Autodesk Fusion 360 part; units mm, degrees
(part 2 of 2)
  spline S289 degree 3 poles (-117.5026, -9.5657) (-117.4851, -9.5569) (-117.4675, -9.5437) (-117.4499, -9.5261) knots 0 0 0 0 1 1 1 1
  spline S290 degree 3 poles (-119.0451, -14.0876) (-119.0187, -13.8591) (-118.9792, -13.6393) (-118.9265, -13.4284) knots 0 0 0 0 1 1 1 1
  line L134 (-80.6655, -26.5854) -> (-81.061, -26.9809)
  spline S291 degree 3 poles (-82.8276, -8.4187) (-82.8627, -8.4187) (-82.9375, -8.3967) (-83.0517, -8.3528) knots 0 0 0 0 1 1 1 1
  line L135 (-81.1665, -9.3679) -> (-82.8276, -8.4187)
  line L136 (-88.7601, -9.2361) -> (-87.9691, -8.7087)
  spline S292 degree 3 poles (-77.8706, -7.575) (-76.6402, -8.4539) (-75.5152, -9.5876) (-74.4957, -10.9763) knots 0 0 0 0 1 1 1 1
  spline S293 degree 3 poles (-118.3332, -11.1081) (-118.0783, -10.3874) (-117.819, -9.8865) (-117.5554, -9.6052) knots 0 0 0 0 1 1 1 1
  line L137 (-77.2115, -23.2368) -> (-80.6655, -26.5854)
  line L138 (-81.7466, -5.9666) -> (-81.6806, -5.9666)
  spline S294 degree 3 poles (-79.9141, -6.4017) (-79.2549, -6.6917) (-78.5738, -7.0828) (-77.8706, -7.575) knots 0 0 0 0 1 1 1 1
  spline S295 degree 3 poles (-81.6147, -5.9666) (-81.1401, -5.9666) (-80.5732, -6.1116) (-79.9141, -6.4017) knots 0 0 0 0 1 1 1 1
  spline S296 degree 3 poles (-72.9664, -15.3795) (-72.9664, -16.4166) (-73.2037, -17.423) (-73.6783, -18.3985) knots 0 0 0 0 1 1 1 1
  line L139 (-92.4251, -25.9262) -> (-92.4251, -21.8921)
  line L140 (-92.4251, -21.8921) -> (-92.4251, -8.3923)
  line L141 (-81.6806, -5.9666) -> (-81.6147, -5.9666)
  spline S297 degree 3 poles (-86.4135, -7.8123) (-85.5522, -7.3377) (-84.7216, -6.9378) (-83.9218, -6.6126) knots 0 0 0 0 1 1 1 1
  spline S298 degree 3 poles (-98.9405, -9.4998) (-99.0108, -9.6052) (-99.0987, -9.7107) (-99.2041, -9.8162) knots 0 0 0 0 1 1 1 1
  spline S299 degree 3 poles (-98.69, -9.1306) (-98.7515, -9.2537) (-98.835, -9.3767) (-98.9405, -9.4998) knots 0 0 0 0 1 1 1 1
  spline S300 degree 3 poles (-76.7896, -16.3024) (-76.7896, -15.1422) (-77.0884, -14.0568) (-77.6861, -13.0461) knots 0 0 0 0 1 1 1 1
  line L142 (-98.5977, -8.7351) -> (-98.5977, -8.7615)
  arc A32 (-108.5643, -6.5335) -> (-108.3534, -6.5467) centre (-108.3531, -4.8477) ccw
  spline S301 degree 3 poles (-112.0711, -8.4714) (-112.4051, -8.4714) (-112.7215, -8.4934) (-113.0203, -8.5374) knots 0 0 0 0 1 1 1 1
  spline S302 degree 3 poles (-104.2665, -9.2625) (-104.3544, -9.2449) (-104.4423, -9.2361) (-104.5302, -9.2361) knots 0 0 0 0 1 1 1 1
  spline S303 degree 3 poles (-101.4321, -11.0422) (-101.4936, -10.8225) (-101.5947, -10.5984) (-101.7353, -10.3699) knots 0 0 0 0 1 1 1 1
  spline S304 degree 3 poles (-110.2518, -8.5769) (-110.5682, -8.5593) (-110.8758, -8.5374) (-111.1746, -8.511) knots 0 0 0 0 1 1 1 1
  line L143 (-76.7896, -16.3683) -> (-76.7896, -16.3024)
  line L144 (-88.7601, -6.573) -> (-88.7601, -9.2361)
  spline S305 degree 3 poles (-119.111, -14.7467) (-119.0934, -14.5358) (-119.0715, -14.3161) (-119.0451, -14.0876) knots 0 0 0 0 1 1 1 1
  spline S306 degree 3 poles (-73.6783, -18.3985) (-74.1529, -19.3741) (-74.6803, -20.2486) (-75.2603, -21.022) knots 0 0 0 0 1 1 1 1
  line L145 (-108.3534, -6.5467) -> (-102.3418, -7.1531)
  spline S307 degree 3 poles (-101.3926, -12.1892) (-101.3574, -12.031) (-101.3398, -11.8728) (-101.3398, -11.7146) knots 0 0 0 0 1 1 1 1
  line L146 (-92.4251, -8.3923) -> (-97.092, -8.3132)
  line L147 (-99.2041, -9.8162) -> (-99.5205, -10.1326)
  spline S308 degree 3 poles (-83.0517, -8.3528) (-83.166, -8.3089) (-83.311, -8.2605) (-83.4868, -8.2078) knots 0 0 0 0 1 1 1 1
  spline S309 degree 3 poles (-104.5302, -9.2361) (-104.6181, -9.2361) (-104.706, -9.2273) (-104.7939, -9.2097) knots 0 0 0 0 1 1 1 1
  line L148 (-100.7598, -11.6882) -> (-100.7861, -11.7146)
  line L149 (-125.9672, -11.385) -> (-125.9672, -11.3191)
  spline S310 degree 3 poles (-101.5508, -12.6901) (-101.4804, -12.5144) (-101.4277, -12.3474) (-101.3926, -12.1892) knots 0 0 0 0 1 1 1 1
  spline S311 degree 3 poles (-101.1553, -12.1892) (-101.2783, -12.3474) (-101.4101, -12.5144) (-101.5508, -12.6901) knots 0 0 0 0 1 1 1 1
  line L150 (-100.7861, -11.7146) -> (-101.1553, -12.1892)
  arc A33 (-166.7633, -25.979) -> (-166.961, -26.0317) centre (-165.2752, -31.9564) ccw
  spline S312 degree 3 poles (-99.9951, -10.6599) (-100.1357, -10.8532) (-100.2632, -11.0246) (-100.3774, -11.174) knots 0 0 0 0 1 1 1 1
  line L151 (-185.9055, -15.2345) -> (-185.9055, -15.2477)
  spline S313 degree 3 poles (-179.9203, -26.4272) (-180.0433, -26.4272) (-180.1708, -26.4228) (-180.3026, -26.414) knots 0 0 0 0 1 1 1 1
  spline S314 degree 3 poles (-187.7644, -20.9693) (-188.6872, -19.7564) (-189.2277, -18.5172) (-189.3859, -17.2516) knots 0 0 0 0 1 1 1 1
  spline S315 degree 3 poles (-175.2534, -7.3377) (-175.2006, -7.3201) (-175.1523, -7.2937) (-175.1084, -7.2586) knots 0 0 0 0 1 1 1 1
  spline S316 degree 3 poles (-189.3859, -17.2516) (-189.4035, -17.1637) (-189.4167, -17.0802) (-189.4255, -17.0011) knots 0 0 0 0 1 1 1 1
  line L152 (-172.3003, -8.7087) -> (-177.0463, -8.656)
  spline S317 degree 3 poles (-166.2623, -25.7417) (-166.3326, -25.7944) (-166.4073, -25.8383) (-166.4864, -25.8735) knots 0 0 0 0 1 1 1 1
  spline S318 degree 3 poles (-99.5205, -10.1326) (-99.6084, -10.2204) (-99.6919, -10.3083) (-99.771, -10.3962) knots 0 0 0 0 1 1 1 1
  line L153 (-186.5911, -10.1853) -> (-185.721, -8.6824)
  spline S319 degree 3 poles (-166.4864, -25.8735) (-166.5655, -25.9087) (-166.6578, -25.9438) (-166.7633, -25.979) knots 0 0 0 0 1 1 1 1
  spline S320 degree 3 poles (-99.7578, -15.3268) (-99.8809, -15.3971) (-100.0479, -15.4894) (-100.2588, -15.6037) knots 0 0 0 0 1 1 1 1
  line L154 (-99.8106, -15.1159) -> (-99.7578, -15.3268)
  spline S321 degree 3 poles (-100.2588, -15.6037) (-100.4697, -15.7179) (-100.707, -15.8278) (-100.9707, -15.9332) knots 0 0 0 0 1 1 1 1
  line L155 (-167.6597, -26.0581) -> (-172.2212, -25.979)
  spline S322 degree 3 poles (-186.7493, -10.4226) (-186.7141, -10.3874) (-186.6834, -10.3479) (-186.657, -10.3039) knots 0 0 0 0 1 1 1 1
  spline S323 degree 3 poles (-188.1994, -7.074) (-187.8127, -6.8982) (-187.593, -6.8016) (-187.5403, -6.784) knots 0 0 0 0 1 1 1 1
  line L156 (-185.721, -8.6824) -> (-190.757, -8.6033)
  spline S324 degree 3 poles (-99.771, -10.3962) (-99.8501, -10.4841) (-99.9248, -10.572) (-99.9951, -10.6599) knots 0 0 0 0 1 1 1 1
  line L157 (-177.0463, -8.656) -> (-175.2534, -7.3377)
  spline S325 degree 3 poles (-175.9916, -25.4253) (-176.6596, -25.7592) (-177.3276, -26.0097) (-177.9955, -26.1767) knots 0 0 0 0 1 1 1 1
  line L158 (-172.3003, -22.1294) -> (-172.3003, -8.7087)
  line L159 (-172.2212, -23.2896) -> (-174.9633, -24.8716)
  line L160 (-172.4321, -22.4195) -> (-172.3003, -22.1294)
  spline S326 degree 3 poles (-179.683, -22.8677) (-179.0326, -23.2193) (-178.3822, -23.4961) (-177.7318, -23.6982) knots 0 0 0 0 1 1 1 1
  spline S327 degree 3 poles (-177.7318, -23.6982) (-177.0815, -23.9004) (-176.4838, -24.0015) (-175.9389, -24.0015) knots 0 0 0 0 1 1 1 1
  spline S328 degree 3 poles (-166.961, -26.0317) (-167.0225, -26.0493) (-167.0797, -26.0581) (-167.1324, -26.0581) knots 0 0 0 0 1 1 1 1
  spline S329 degree 3 poles (-189.465, -7.7332) (-189.008, -7.4695) (-188.5862, -7.2498) (-188.1994, -7.074) knots 0 0 0 0 1 1 1 1
  spline S330 degree 3 poles (-190.1506, -8.155) (-189.9221, -7.9968) (-189.6936, -7.8562) (-189.465, -7.7332) knots 0 0 0 0 1 1 1 1
  line L161 (-189.4387, -16.6979) -> (-189.4387, -16.6451)
  line L162 (-189.4387, -16.777) -> (-189.4387, -16.6979)
  spline S331 degree 3 poles (-100.7334, -11.6355) (-100.7334, -11.653) (-100.7422, -11.6706) (-100.7598, -11.6882) knots 0 0 0 0 1 1 1 1
  spline S332 degree 3 poles (-180.7113, -26.3745) (-181.1332, -26.3217) (-181.7132, -26.0932) (-182.4515, -25.6889) knots 0 0 0 0 1 1 1 1
  spline S333 degree 3 poles (-189.4387, -16.6451) (-189.4387, -15.6608) (-189.1574, -14.6588) (-188.5949, -13.6393) knots 0 0 0 0 1 1 1 1
  spline S334 degree 3 poles (-184.7454, -24.1069) (-185.8352, -23.228) (-186.8416, -22.1822) (-187.7644, -20.9693) knots 0 0 0 0 1 1 1 1
  arc A34 (-100.7334, -11.6355) -> (-100.3774, -11.174) centre (-156.8917, 32.0547) ccw
  spline S335 degree 3 poles (-177.9955, -26.1767) (-178.6635, -26.3437) (-179.3051, -26.4272) (-179.9203, -26.4272) knots 0 0 0 0 1 1 1 1
  line L163 (-185.9055, -15.195) -> (-185.9055, -15.2345)
  spline S336 degree 3 poles (-174.9633, -24.8716) (-175.1391, -24.9946) (-175.3105, -25.1001) (-175.4775, -25.188) knots 0 0 0 0 1 1 1 1
  line L164 (-167.5015, -26.0581) -> (-167.5675, -26.0581)
  spline S337 degree 3 poles (-186.657, -10.3039) (-186.6306, -10.26) (-186.6086, -10.2204) (-186.5911, -10.1853) knots 0 0 0 0 1 1 1 1
  line L165 (-185.9055, -15.2477) -> (-185.9055, -15.2213)
  spline S338 degree 3 poles (-100.9707, -15.9332) (-101.1816, -16.0387) (-101.4057, -16.1354) (-101.643, -16.2233) knots 0 0 0 0 1 1 1 1
  spline S339 degree 3 poles (-180.3026, -26.414) (-180.4344, -26.4052) (-180.5707, -26.3921) (-180.7113, -26.3745) knots 0 0 0 0 1 1 1 1
  line L166 (-167.5675, -26.0581) -> (-167.6597, -26.0581)
  spline S340 degree 3 poles (-188.5949, -13.6393) (-188.0325, -12.6198) (-187.4172, -11.5476) (-186.7493, -10.4226) knots 0 0 0 0 1 1 1 1
  spline S341 degree 3 poles (-189.4255, -17.0011) (-189.4343, -16.922) (-189.4387, -16.8473) (-189.4387, -16.777) knots 0 0 0 0 1 1 1 1
  line L167 (-172.2212, -25.979) -> (-172.2212, -23.2896)
  line L168 (-167.317, -26.0581) -> (-167.5015, -26.0581)
  arc A35 (-175.9916, -25.4253) -> (-175.4775, -25.188) centre (-178.0133, -20.3693) ccw
  arc A36 (-102.3681, -16.4606) -> (-101.643, -16.2233) centre (-105.1088, -6.8599) ccw
  spline S342 degree 3 poles (-175.1084, -7.2586) (-175.0644, -7.2234) (-175.0161, -7.1883) (-174.9633, -7.1531) knots 0 0 0 0 1 1 1 1
  spline S343 degree 3 poles (-172.9858, -23.0786) (-172.7046, -22.8325) (-172.52, -22.6128) (-172.4321, -22.4195) knots 0 0 0 0 1 1 1 1
  spline S344 degree 3 poles (-182.4515, -25.6889) (-183.1898, -25.2846) (-183.9544, -24.7573) (-184.7454, -24.1069) knots 0 0 0 0 1 1 1 1
  spline S345 degree 3 poles (-190.757, -8.6033) (-190.5812, -8.4627) (-190.3791, -8.3132) (-190.1506, -8.155) knots 0 0 0 0 1 1 1 1
  line L169 (-167.1324, -26.0581) -> (-167.317, -26.0581)
  line L170 (-175.9389, -24.0015) -> (-175.8862, -24.0015)
  spline S346 degree 3 poles (-174.0141, -23.6719) (-173.5747, -23.4873) (-173.2319, -23.2896) (-172.9858, -23.0786) knots 0 0 0 0 1 1 1 1
  line L171 (-175.7807, -24.0015) -> (-175.728, -24.0015)
  line L172 (-175.8862, -24.0015) -> (-175.8334, -24.0015)
  spline S347 degree 3 poles (-175.728, -24.0015) (-175.0249, -23.9663) (-174.4536, -23.8564) (-174.0141, -23.6719) knots 0 0 0 0 1 1 1 1
  line L173 (-175.8334, -24.0015) -> (-175.7807, -24.0015)
  spline S348 degree 3 poles (-183.4007, -20.1124) (-182.2406, -21.2637) (-181.0013, -22.1822) (-179.683, -22.8677) knots 0 0 0 0 1 1 1 1
  spline S349 degree 3 poles (-174.9633, -7.1531) (-174.8754, -7.1004) (-174.7832, -7.0476) (-174.6865, -6.9949) knots 0 0 0 0 1 1 1 1
  line L174 (-173.4341, -6.7049) -> (-168.6353, -6.6785)
  arc A37 (-174.3833, -6.8631) -> (-174.6865, -6.9949) centre (-173.796, -8.6285) ccw
  line L175 (-200.4961, -12.2155) -> (-200.4961, -12.0573)
  spline S350 degree 3 poles (-173.9614, -6.7576) (-173.8911, -6.74) (-173.812, -6.7268) (-173.7241, -6.7181) knots 0 0 0 0 1 1 1 1
  spline S351 degree 3 poles (-206.6263, -17.067) (-206.5824, -17.0494) (-206.5428, -17.0319) (-206.5077, -17.0143) knots 0 0 0 0 1 1 1 1
  spline S352 degree 3 poles (-207.5887, -8.1814) (-207.7469, -8.199) (-207.9095, -8.2254) (-208.0765, -8.2605) knots 0 0 0 0 1 1 1 1
  spline S353 degree 3 poles (-166.17, -25.6889) (-166.1964, -25.7065) (-166.2271, -25.7241) (-166.2623, -25.7417) knots 0 0 0 0 1 1 1 1
  spline S354 degree 3 poles (-205.1762, -16.5265) (-205.0619, -16.4825) (-204.952, -16.4342) (-204.8466, -16.3815) knots 0 0 0 0 1 1 1 1
  spline S355 degree 3 poles (-206.6, -8.1814) (-206.6439, -8.1814) (-206.6835, -8.1726) (-206.7186, -8.155) knots 0 0 0 0 1 1 1 1
  spline S356 degree 3 poles (-200.4961, -12.0573) (-200.4961, -12.0046) (-200.5049, -11.9606) (-200.5224, -11.9255) knots 0 0 0 0 1 1 1 1
  spline S357 degree 3 poles (-195.2623, -25.1616) (-195.4293, -25.2671) (-195.5918, -25.3637) (-195.75, -25.4516) knots 0 0 0 0 1 1 1 1
  spline S358 degree 3 poles (-166.1041, -25.6098) (-166.1217, -25.645) (-166.1437, -25.6714) (-166.17, -25.6889) knots 0 0 0 0 1 1 1 1
  spline S359 degree 3 poles (-202.8954, -15.2609) (-202.2626, -14.8127) (-201.7441, -14.3512) (-201.3398, -13.8766) knots 0 0 0 0 1 1 1 1
  spline S360 degree 3 poles (-206.745, -17.1197) (-206.7098, -17.1022) (-206.6703, -17.0846) (-206.6263, -17.067) knots 0 0 0 0 1 1 1 1
  spline S361 degree 3 poles (-207.2855, -8.1682) (-207.3822, -8.177) (-207.4833, -8.1814) (-207.5887, -8.1814) knots 0 0 0 0 1 1 1 1
  spline S362 degree 3 poles (-208.0765, -8.2605) (-208.2435, -8.2957) (-208.4237, -8.3308) (-208.617, -8.366) knots 0 0 0 0 1 1 1 1
  spline S363 degree 3 poles (-195.75, -25.4516) (-196.0664, -25.6098) (-196.3916, -25.7417) (-196.7256, -25.8471) knots 0 0 0 0 1 1 1 1
  spline S364 degree 3 poles (-193.878, -24.397) (-194.0362, -24.4849) (-194.1856, -24.564) (-194.3262, -24.6343) knots 0 0 0 0 1 1 1 1
  line L176 (-164.2321, -24.186) -> (-166.1041, -25.6098)
  arc A38 (-194.7481, -24.8716) -> (-195.2623, -25.1616) centre (-192.0994, -30.1677) ccw
  spline S365 degree 3 poles (-205.5057, -16.6188) (-205.4003, -16.6012) (-205.2904, -16.5704) (-205.1762, -16.5265) knots 0 0 0 0 1 1 1 1
  spline S366 degree 3 poles (-205.5848, -19.3082) (-205.954, -18.8687) (-206.2836, -18.4601) (-206.5736, -18.0821) knots 0 0 0 0 1 1 1 1
  spline S367 degree 3 poles (-207.035, -17.3307) (-207.0174, -17.2779) (-206.9823, -17.234) (-206.9296, -17.1988) knots 0 0 0 0 1 1 1 1
  line L177 (-206.5077, -17.0143) -> (-205.5057, -16.6188)
  spline S368 degree 3 poles (-192.5333, -23.3555) (-192.3927, -23.2764) (-192.3136, -23.2368) (-192.296, -23.2368) knots 0 0 0 0 1 1 1 1
  spline S369 degree 3 poles (-204.8466, -16.3815) (-204.1786, -16.0827) (-203.5282, -15.7091) (-202.8954, -15.2609) knots 0 0 0 0 1 1 1 1
  spline S370 degree 3 poles (-194.3262, -24.6343) (-194.4669, -24.7046) (-194.6075, -24.7837) (-194.7481, -24.8716) knots 0 0 0 0 1 1 1 1
  spline S371 degree 3 poles (-185.8528, -15.9332) (-185.8176, -16.1442) (-185.7737, -16.3463) (-185.721, -16.5397) knots 0 0 0 0 1 1 1 1
  line L178 (-185.9055, -15.2213) -> (-185.9319, -15.3004)
  line L179 (-168.5035, -24.0278) -> (-164.2321, -24.186)
  spline S372 degree 3 poles (-205.5189, -19.3873) (-205.5453, -19.3521) (-205.5673, -19.3258) (-205.5848, -19.3082) knots 0 0 0 0 1 1 1 1
  spline S373 degree 3 poles (-206.5736, -18.0821) (-206.8636, -17.7042) (-207.0174, -17.4625) (-207.035, -17.357) knots 0 0 0 0 1 1 1 1
  line L180 (-206.8636, -8.155) -> (-206.9823, -8.155)
  spline S374 degree 3 poles (-202.7109, -9.1438) (-203.8534, -8.5725) (-205.1015, -8.2517) (-206.4549, -8.1814) knots 0 0 0 0 1 1 1 1
  line L181 (-192.296, -23.2368) -> (-192.1114, -23.5532)
  line L182 (-206.4549, -8.1814) -> (-206.6, -8.1814)
  line L183 (-174.3833, -6.8631) -> (-174.1723, -6.8103)
  spline S375 degree 3 poles (-200.5224, -11.9255) (-200.8388, -10.6423) (-201.5683, -9.7151) (-202.7109, -9.1438) knots 0 0 0 0 1 1 1 1
  spline S376 degree 3 poles (-196.7256, -25.8471) (-197.0596, -25.9526) (-197.4287, -26.0053) (-197.833, -26.0053) knots 0 0 0 0 1 1 1 1
  line L184 (-192.1114, -23.5532) -> (-193.878, -24.397)
  line L185 (-168.6353, -6.6785) -> (-168.5826, -10.5281)
  line L186 (-168.5826, -10.5281) -> (-168.5035, -24.0278)
  spline S377 degree 3 poles (-206.9823, -8.155) (-207.0878, -8.155) (-207.1888, -8.1594) (-207.2855, -8.1682) knots 0 0 0 0 1 1 1 1
  spline S378 degree 3 poles (-193.0606, -23.606) (-192.8497, -23.5181) (-192.6739, -23.4346) (-192.5333, -23.3555) knots 0 0 0 0 1 1 1 1
  spline S379 degree 3 poles (-173.7241, -6.7181) (-173.6362, -6.7093) (-173.5395, -6.7049) (-173.4341, -6.7049) knots 0 0 0 0 1 1 1 1
  spline S380 degree 3 poles (-206.9296, -17.1988) (-206.8768, -17.1637) (-206.8153, -17.1373) (-206.745, -17.1197) knots 0 0 0 0 1 1 1 1
  spline S381 degree 3 poles (-186.2483, -6.6785) (-186.0549, -6.6785) (-185.8484, -6.6829) (-185.6287, -6.6917) knots 0 0 0 0 1 1 1 1
  spline S382 degree 3 poles (-185.6287, -6.6917) (-185.409, -6.7005) (-185.1848, -6.7049) (-184.9563, -6.7049) knots 0 0 0 0 1 1 1 1
  spline S383 degree 3 poles (-187.0129, -6.7049) (-186.7844, -6.6873) (-186.5295, -6.6785) (-186.2483, -6.6785) knots 0 0 0 0 1 1 1 1
  spline S384 degree 3 poles (-153.2463, -6.4148) (-152.9739, -6.4324) (-152.6883, -6.4588) (-152.3894, -6.4939) knots 0 0 0 0 1 1 1 1
  spline S385 degree 3 poles (-187.5403, -6.784) (-187.4172, -6.7488) (-187.2415, -6.7225) (-187.0129, -6.7049) knots 0 0 0 0 1 1 1 1
  spline S386 degree 3 poles (-200.7202, -13.0197) (-200.5708, -12.7297) (-200.4961, -12.4616) (-200.4961, -12.2155) knots 0 0 0 0 1 1 1 1
  spline S387 degree 3 poles (-185.721, -16.5397) (-185.3343, -17.7701) (-184.5608, -18.961) (-183.4007, -20.1124) knots 0 0 0 0 1 1 1 1
  line L187 (-206.7186, -8.155) -> (-206.8636, -8.155)
  line L188 (-154.2483, -6.3885) -> (-153.9978, -6.3885)
  spline S388 degree 3 poles (-153.9978, -6.3885) (-153.7693, -6.3885) (-153.5188, -6.3973) (-153.2463, -6.4148) knots 0 0 0 0 1 1 1 1
  spline S389 degree 3 poles (-154.4724, -6.4148) (-154.4021, -6.3973) (-154.3274, -6.3885) (-154.2483, -6.3885) knots 0 0 0 0 1 1 1 1
  line L189 (-174.1723, -6.8103) -> (-173.9614, -6.7576)
  line L190 (-207.035, -17.357) -> (-207.035, -17.3307)
  line L191 (-197.833, -26.0053) -> (-197.8989, -26.0053)
  spline S390 degree 3 poles (-201.3398, -13.8766) (-201.0761, -13.5954) (-200.8696, -13.3097) (-200.7202, -13.0197) knots 0 0 0 0 1 1 1 1
  arc A39 (-185.9319, -15.3004) -> (-185.8528, -15.9332) centre (-178.1834, -14.6532) ccw
  line L192 (-208.617, -8.366) -> (-208.617, -8.3396)
  spline S391 degree 3 poles (-146.2196, -16.5133) (-147.1688, -16.7242) (-148.1664, -16.8649) (-149.2122, -16.9352) knots 0 0 0 0 1 1 1 1
  spline S392 degree 3 poles (-143.873, -15.6037) (-144.0839, -15.7179) (-144.3212, -15.8278) (-144.5849, -15.9332) knots 0 0 0 0 1 1 1 1
  line L193 (-143.4247, -15.1159) -> (-143.372, -15.3268)
  arc A40 (-144.3476, -11.6355) -> (-143.9916, -11.174) centre (-200.5059, 32.0547) ccw
  line L194 (-142.8183, -9.8162) -> (-143.1347, -10.1326)
  spline S393 degree 3 poles (-145.3495, -10.3699) (-145.6132, -9.9128) (-145.9735, -9.6228) (-146.4305, -9.4998) knots 0 0 0 0 1 1 1 1
  line L195 (-144.3739, -11.6882) -> (-144.4003, -11.7146)
  spline S394 degree 3 poles (-145.2968, -7.2586) (-144.9276, -7.3113) (-144.5233, -7.3992) (-144.0839, -7.5222) knots 0 0 0 0 1 1 1 1
  arc A41 (-184.7981, -11.5564) -> (-184.429, -10.8049) centre (-238.7282, 15.402) ccw
  line L196 (-144.4003, -11.7146) -> (-144.7694, -12.1892)
  spline S395 degree 3 poles (-158.6647, -8.6824) (-158.4538, -8.6121) (-158.2428, -8.533) (-158.0319, -8.4451) knots 0 0 0 0 1 1 1 1
  line L197 (-185.9055, -15.1422) -> (-185.9055, -15.1554)
  spline S396 degree 3 poles (-185.576, -13.5207) (-185.7957, -14.1623) (-185.9055, -14.7028) (-185.9055, -15.1422) knots 0 0 0 0 1 1 1 1
  spline S397 degree 3 poles (-147.8807, -9.2625) (-147.9686, -9.2449) (-148.0565, -9.2361) (-148.1444, -9.2361) knots 0 0 0 0 1 1 1 1
  spline S398 degree 3 poles (-155.6853, -8.4714) (-156.0193, -8.4714) (-156.3357, -8.4934) (-156.6345, -8.5374) knots 0 0 0 0 1 1 1 1
  spline S399 degree 3 poles (-145.9823, -16.4606) (-146.0175, -16.4606) (-146.057, -16.465) (-146.101, -16.4738) knots 0 0 0 0 1 1 1 1
  spline S400 degree 3 poles (-144.0839, -7.5222) (-143.6269, -7.6453) (-143.205, -7.8035) (-142.8183, -7.9968) knots 0 0 0 0 1 1 1 1
  spline S401 degree 3 poles (-156.2917, -7.4695) (-155.9402, -7.2234) (-155.6106, -6.9905) (-155.303, -6.7708) knots 0 0 0 0 1 1 1 1
  spline S402 degree 3 poles (-144.3476, -11.6355) (-144.3476, -11.653) (-144.3564, -11.6706) (-144.3739, -11.6882) knots 0 0 0 0 1 1 1 1
  spline S403 degree 3 poles (-158.5065, -17.1197) (-158.3132, -17.4361) (-158.0363, -17.8053) (-157.676, -18.2271) knots 0 0 0 0 1 1 1 1
  spline S404 degree 3 poles (-146.4305, -9.4998) (-146.8876, -9.3767) (-147.371, -9.2976) (-147.8807, -9.2625) knots 0 0 0 0 1 1 1 1
  spline S405 degree 3 poles (-184.7981, -11.5564) (-185.097, -12.2243) (-185.3562, -12.8791) (-185.576, -13.5207) knots 0 0 0 0 1 1 1 1
  spline S406 degree 3 poles (-144.5849, -15.9332) (-144.7958, -16.0387) (-145.0199, -16.1354) (-145.2572, -16.2233) knots 0 0 0 0 1 1 1 1
  spline S407 degree 3 poles (-158.0319, -8.4451) (-157.821, -8.3572) (-157.6188, -8.2693) (-157.4255, -8.1814) knots 0 0 0 0 1 1 1 1
  spline S408 degree 3 poles (-144.954, -11.7146) (-144.954, -11.486) (-144.9848, -11.2619) (-145.0463, -11.0422) knots 0 0 0 0 1 1 1 1
  spline S409 degree 3 poles (-182.1878, -6.9422) (-182.223, -6.9598) (-182.4295, -7.2762) (-182.8074, -7.8914) knots 0 0 0 0 1 1 1 1
  line L198 (-151.9676, -6.5467) -> (-145.9559, -7.1531)
  spline S410 degree 3 poles (-145.1649, -12.6901) (-145.0946, -12.5144) (-145.0419, -12.3474) (-145.0067, -12.1892) knots 0 0 0 0 1 1 1 1
  spline S411 degree 3 poles (-145.0463, -11.0422) (-145.1078, -10.8225) (-145.2089, -10.5984) (-145.3495, -10.3699) knots 0 0 0 0 1 1 1 1
  spline S412 degree 3 poles (-182.8074, -7.8914) (-183.1854, -8.5066) (-183.5941, -9.2361) (-184.0335, -10.0798) knots 0 0 0 0 1 1 1 1
  spline S413 degree 3 poles (-184.0335, -10.0798) (-184.1741, -10.3083) (-184.306, -10.55) (-184.429, -10.8049) knots 0 0 0 0 1 1 1 1
  arc A42 (-183.5062, -6.8103) -> (-184.2181, -6.7576) centre (-193.5222, -137.1956) ccw
  line L199 (-184.9563, -6.7049) -> (-184.2181, -6.7576)
  spline S414 degree 3 poles (-182.5965, -6.9026) (-182.3416, -6.929) (-182.2054, -6.9422) (-182.1878, -6.9422) knots 0 0 0 0 1 1 1 1
  spline S415 degree 3 poles (-142.8183, -7.9968) (-142.4316, -8.1902) (-142.2294, -8.4363) (-142.2119, -8.7351) knots 0 0 0 0 1 1 1 1
  arc A43 (-145.9823, -16.4606) -> (-145.2572, -16.2233) centre (-148.723, -6.8599) ccw
  spline S416 degree 3 poles (-142.5546, -9.4998) (-142.6249, -9.6052) (-142.7128, -9.7107) (-142.8183, -9.8162) knots 0 0 0 0 1 1 1 1
  line L200 (-161.0641, -9.4998) -> (-161.1168, -9.5261)
  spline S417 degree 3 poles (-143.372, -15.3268) (-143.495, -15.3971) (-143.662, -15.4894) (-143.873, -15.6037) knots 0 0 0 0 1 1 1 1
  spline S418 degree 3 poles (-142.2119, -8.7615) (-142.2119, -8.8845) (-142.2426, -9.0076) (-142.3041, -9.1306) knots 0 0 0 0 1 1 1 1
  spline S419 degree 3 poles (-148.1444, -9.2361) (-148.2323, -9.2361) (-148.3202, -9.2273) (-148.408, -9.2097) knots 0 0 0 0 1 1 1 1
  line L201 (-185.9055, -15.1554) -> (-185.9055, -15.195)
  spline S420 degree 3 poles (-143.8598, -15.2477) (-143.7279, -15.2125) (-143.5829, -15.1686) (-143.4247, -15.1159) knots 0 0 0 0 1 1 1 1
  spline S421 degree 3 poles (-143.3852, -10.3962) (-143.4643, -10.4841) (-143.539, -10.572) (-143.6093, -10.6599) knots 0 0 0 0 1 1 1 1
  spline S422 degree 3 poles (-160.2467, -9.2229) (-159.7545, -9.0735) (-159.2272, -8.8933) (-158.6647, -8.6824) knots 0 0 0 0 1 1 1 1
  spline S423 degree 3 poles (-142.3041, -9.1306) (-142.3657, -9.2537) (-142.4492, -9.3767) (-142.5546, -9.4998) knots 0 0 0 0 1 1 1 1
  line L202 (-142.2119, -8.7351) -> (-142.2119, -8.7615)
  spline S424 degree 3 poles (-161.1168, -9.5261) (-161.0289, -9.4734) (-160.7389, -9.3723) (-160.2467, -9.2229) knots 0 0 0 0 1 1 1 1
  arc A44 (-152.1785, -6.5335) -> (-151.9676, -6.5467) centre (-151.9673, -4.8477) ccw
  arc A45 (-154.7888, -8.511) -> (-155.6853, -8.4714) centre (-155.6859, -18.666) ccw
  spline S425 degree 3 poles (-143.1347, -10.1326) (-143.2226, -10.2204) (-143.3061, -10.3083) (-143.3852, -10.3962) knots 0 0 0 0 1 1 1 1
  spline S426 degree 3 poles (-145.9559, -7.1531) (-145.8856, -7.1707) (-145.6659, -7.2058) (-145.2968, -7.2586) knots 0 0 0 0 1 1 1 1
  spline S427 degree 3 poles (-153.866, -8.5769) (-154.1824, -8.5593) (-154.49, -8.5374) (-154.7888, -8.511) knots 0 0 0 0 1 1 1 1
  spline S428 degree 3 poles (-157.4255, -8.1814) (-157.2321, -8.0759) (-157.0388, -7.9617) (-156.8454, -7.8386) knots 0 0 0 0 1 1 1 1
  line L203 (-152.6531, -17.067) -> (-158.5065, -17.1197)
  spline S429 degree 3 poles (-143.6093, -10.6599) (-143.7499, -10.8532) (-143.8774, -11.0246) (-143.9916, -11.174) knots 0 0 0 0 1 1 1 1
  line L204 (-148.408, -9.2097) -> (-153.866, -8.5769)
  spline S430 degree 3 poles (-149.2122, -16.9352) (-150.2581, -17.0055) (-151.4051, -17.0494) (-152.6531, -17.067) knots 0 0 0 0 1 1 1 1
  spline S431 degree 3 poles (-145.0067, -12.1892) (-144.9716, -12.031) (-144.954, -11.8728) (-144.954, -11.7146) knots 0 0 0 0 1 1 1 1
  arc A46 (-152.3894, -6.4939) -> (-152.1785, -6.5335) centre (-151.9567, -4.7686) ccw
  spline S432 degree 3 poles (-155.303, -6.7708) (-154.9953, -6.5511) (-154.7185, -6.4324) (-154.4724, -6.4148) knots 0 0 0 0 1 1 1 1
  spline S433 degree 3 poles (-156.8454, -7.8386) (-156.6521, -7.7156) (-156.4675, -7.5926) (-156.2917, -7.4695) knots 0 0 0 0 1 1 1 1
  spline S434 degree 3 poles (-146.101, -16.4738) (-146.1449, -16.4825) (-146.1845, -16.4957) (-146.2196, -16.5133) knots 0 0 0 0 1 1 1 1
  spline S435 degree 3 poles (-144.7694, -12.1892) (-144.8925, -12.3474) (-145.0243, -12.5144) (-145.1649, -12.6901) knots 0 0 0 0 1 1 1 1
  arc A47 (-144.2685, -15.3532) -> (-143.8598, -15.2477) centre (-150.819, 10.8745) ccw
  line L205 (-122.5131, -9.7898) -> (-122.5131, -9.8425)
  spline S436 degree 3 poles (-143.6357, -22.2876) (-143.6884, -22.3755) (-143.7587, -22.4634) (-143.8466, -22.5513) knots 0 0 0 0 1 1 1 1
  line L206 (-151.1238, -25.979) -> (-151.282, -25.979)
  line L207 (-127.1009, -14.1667) -> (-125.9408, -14.404)
  line L208 (-144.5058, -23.0523) -> (-147.7489, -25.0561)
  spline S437 degree 3 poles (-124.1479, -7.2322) (-123.1283, -7.8299) (-122.5834, -8.6648) (-122.5131, -9.7371) knots 0 0 0 0 1 1 1 1
  line L209 (-122.5131, -9.8953) -> (-122.5131, -9.948)
  spline S438 degree 3 poles (-151.6775, -22.7886) (-151.1326, -23.0523) (-150.5833, -23.2588) (-150.0296, -23.4082) knots 0 0 0 0 1 1 1 1
  spline S439 degree 3 poles (-144.0839, -22.7622) (-144.1718, -22.8325) (-144.2597, -22.8941) (-144.3476, -22.9468) knots 0 0 0 0 1 1 1 1
  spline S440 degree 3 poles (-149.911, -25.8735) (-150.2625, -25.9262) (-150.6668, -25.9614) (-151.1238, -25.979) knots 0 0 0 0 1 1 1 1
  spline S441 degree 3 poles (-123.5414, -12.2683) (-124.227, -12.8659) (-125.0268, -13.3493) (-125.9408, -13.7184) knots 0 0 0 0 1 1 1 1
  line L210 (-122.5131, -9.7371) -> (-122.5131, -9.7898)
  spline S442 degree 3 poles (-152.8245, -22.1953) (-152.4466, -22.4151) (-152.0642, -22.6128) (-151.6775, -22.7886) knots 0 0 0 0 1 1 1 1
  line L211 (-162.7516, -15.5905) -> (-162.7516, -15.1686)
  spline S443 degree 3 poles (-158.5197, -10.1853) (-158.8097, -10.9587) (-159.0163, -11.7937) (-159.1393, -12.6901) knots 0 0 0 0 1 1 1 1
  line L212 (-120.7465, -18.8995) -> (-120.7465, -18.9654)
  spline S444 degree 3 poles (-147.5116, -23.5928) (-147.2479, -23.5664) (-146.9755, -23.5269) (-146.6942, -23.4741) knots 0 0 0 0 1 1 1 1
  spline S445 degree 3 poles (-143.5566, -22.0503) (-143.5566, -22.1206) (-143.5829, -22.1997) (-143.6357, -22.2876) knots 0 0 0 0 1 1 1 1
  spline S446 degree 3 poles (-122.4208, -15.8937) (-121.375, -16.6056) (-120.8169, -17.5856) (-120.7465, -18.8336) knots 0 0 0 0 1 1 1 1
  spline S447 degree 3 poles (-154.4724, -25.3462) (-154.8767, -25.188) (-155.2766, -24.9902) (-155.6721, -24.7529) knots 0 0 0 0 1 1 1 1
  spline S448 degree 3 poles (-145.7977, -15.6037) (-145.5868, -15.5773) (-145.3583, -15.5465) (-145.1122, -15.5114) knots 0 0 0 0 1 1 1 1
  line L213 (-159.2975, -15.2213) -> (-147.828, -15.6168)
  spline S449 degree 3 poles (-144.3476, -22.9468) (-144.3651, -22.9644) (-144.3871, -22.982) (-144.4135, -22.9995) knots 0 0 0 0 1 1 1 1
  line L214 (-156.819, -23.9487) -> (-159.904, -21.4175)
  spline S450 degree 3 poles (-144.4135, -22.9995) (-144.4399, -23.0171) (-144.4706, -23.0347) (-144.5058, -23.0523) knots 0 0 0 0 1 1 1 1
  spline S451 degree 3 poles (-122.5131, -9.948) (-122.5131, -10.8972) (-122.8559, -11.6706) (-123.5414, -12.2683) knots 0 0 0 0 1 1 1 1
  spline S452 degree 3 poles (-143.8466, -22.5513) (-143.9169, -22.6216) (-143.996, -22.6919) (-144.0839, -22.7622) knots 0 0 0 0 1 1 1 1
  line L215 (-122.5131, -9.8425) -> (-122.5131, -9.8953)
  spline S453 degree 3 poles (-125.9408, -14.404) (-124.64, -14.6852) (-123.4667, -15.1818) (-122.4208, -15.8937) knots 0 0 0 0 1 1 1 1
  spline S454 degree 3 poles (-143.9784, -22.1953) (-143.6972, -22.0284) (-143.5566, -21.98) (-143.5566, -22.0503) knots 0 0 0 0 1 1 1 1
  spline S455 degree 3 poles (-146.6942, -23.4741) (-146.5536, -23.439) (-146.3998, -23.395) (-146.2328, -23.3423) knots 0 0 0 0 1 1 1 1
  spline S456 degree 3 poles (-162.066, -18.8468) (-162.523, -17.9064) (-162.7516, -16.8209) (-162.7516, -15.5905) knots 0 0 0 0 1 1 1 1
  spline S457 degree 3 poles (-159.904, -21.4175) (-160.8883, -20.6441) (-161.609, -19.7872) (-162.066, -18.8468) knots 0 0 0 0 1 1 1 1
  spline S458 degree 3 poles (-152.9036, -25.834) (-153.4221, -25.7373) (-153.9451, -25.5747) (-154.4724, -25.3462) knots 0 0 0 0 1 1 1 1
  line L216 (-120.7465, -19.0445) -> (-120.7465, -19.1236)
  spline S459 degree 3 poles (-145.1122, -15.5114) (-144.954, -15.4762) (-144.8046, -15.4455) (-144.664, -15.4191) knots 0 0 0 0 1 1 1 1
  arc A48 (-146.2328, -23.3423) -> (-145.745, -23.1577) centre (-147.6288, -18.9161) ccw
  line L217 (-146.7074, -15.6432) -> (-146.4042, -15.6432)
  line L218 (-159.2448, -13.9294) -> (-159.2975, -15.2213)
  arc A49 (-147.828, -15.6168) -> (-147.4061, -15.6432) centre (-147.4055, -12.2452) ccw
  spline S460 degree 3 poles (-148.8563, -25.6098) (-149.2078, -25.7329) (-149.5594, -25.8208) (-149.911, -25.8735) knots 0 0 0 0 1 1 1 1
  line L219 (-147.4061, -15.6432) -> (-147.0106, -15.6432)
  line L220 (-125.9408, -13.7184) -> (-127.1009, -14.1667)
  spline S461 degree 3 poles (-147.7489, -25.0561) (-147.9422, -25.1968) (-148.1312, -25.311) (-148.3158, -25.3989) knots 0 0 0 0 1 1 1 1
  spline S462 degree 3 poles (-148.2762, -23.6323) (-148.0301, -23.6323) (-147.7752, -23.6191) (-147.5116, -23.5928) knots 0 0 0 0 1 1 1 1
  line L221 (-147.0106, -15.6432) -> (-146.7074, -15.6432)
  spline S463 degree 3 poles (-156.6345, -8.5374) (-156.9333, -8.5813) (-157.2321, -8.6648) (-157.5309, -8.7878) knots 0 0 0 0 1 1 1 1
  line L222 (-120.7465, -18.9654) -> (-120.7465, -19.0445)
  spline S464 degree 3 poles (-145.3627, -22.96) (-145.2309, -22.8985) (-145.1034, -22.8325) (-144.9804, -22.7622) knots 0 0 0 0 1 1 1 1
  spline S465 degree 3 poles (-145.745, -23.1577) (-145.622, -23.0874) (-145.4945, -23.0215) (-145.3627, -22.96) knots 0 0 0 0 1 1 1 1
  spline S466 degree 3 poles (-150.0296, -23.4082) (-149.4759, -23.5576) (-148.8914, -23.6323) (-148.2762, -23.6323) knots 0 0 0 0 1 1 1 1
  spline S467 degree 3 poles (-155.6721, -24.7529) (-156.0676, -24.5156) (-156.4499, -24.2476) (-156.819, -23.9487) knots 0 0 0 0 1 1 1 1
  spline S468 degree 3 poles (-151.4402, -25.979) (-151.8972, -25.979) (-152.385, -25.9306) (-152.9036, -25.834) knots 0 0 0 0 1 1 1 1
  spline S469 degree 3 poles (-183.5062, -6.8103) (-183.1546, -6.8455) (-182.8514, -6.8763) (-182.5965, -6.9026) knots 0 0 0 0 1 1 1 1
  line L223 (-151.282, -25.979) -> (-151.4402, -25.979)
  spline S470 degree 3 poles (-148.3158, -25.3989) (-148.5003, -25.4868) (-148.6805, -25.5571) (-148.8563, -25.6098) knots 0 0 0 0 1 1 1 1
  spline S471 degree 3 poles (-144.664, -15.4191) (-144.5233, -15.3927) (-144.3915, -15.3707) (-144.2685, -15.3532) knots 0 0 0 0 1 1 1 1
  spline S472 degree 3 poles (-159.2184, -13.3229) (-159.236, -13.5339) (-159.2448, -13.736) (-159.2448, -13.9294) knots 0 0 0 0 1 1 1 1
  spline S473 degree 3 poles (-144.9804, -22.7622) (-144.5937, -22.5513) (-144.2597, -22.3623) (-143.9784, -22.1953) knots 0 0 0 0 1 1 1 1
  spline S474 degree 3 poles (-146.4042, -15.6432) (-146.2108, -15.6432) (-146.0087, -15.63) (-145.7977, -15.6037) knots 0 0 0 0 1 1 1 1
  line L224 (-120.7465, -18.8336) -> (-120.7465, -18.8995)
  spline S475 degree 3 poles (-120.7465, -19.1236) (-120.729, -20.9693) (-121.7001, -22.4414) (-123.6601, -23.54) knots 0 0 0 0 1 1 1 1
  arc A50 (-159.1393, -12.6901) -> (-159.2184, -13.3229) centre (-151.4699, -13.9702) ccw
  spline S476 degree 3 poles (-16.6417, -26.9018) (-16.6417, -26.8842) (-16.6373, -26.871) (-16.6285, -26.8623) knots 0 0 0 0 1 1 1 1
  spline S477 degree 3 poles (-15.6398, -26.9809) (-15.798, -27.1391) (-15.9737, -27.2973) (-16.1671, -27.4555) knots 0 0 0 0 1 1 1 1
  spline S478 degree 3 poles (-44.8969, -6.2698) (-44.352, -6.1556) (-43.7632, -6.0984) (-43.1304, -6.0984) knots 0 0 0 0 1 1 1 1
  spline S479 degree 3 poles (-53.9407, -16.0783) (-53.9232, -15.7882) (-53.888, -15.5026) (-53.8353, -15.2213) knots 0 0 0 0 1 1 1 1
  line L225 (-68.4206, -20.8902) -> (-68.4734, -20.9957)
  line L226 (-16.2726, -27.561) -> (-16.378, -27.6664)
  line L227 (-11.7902, -23.2368) -> (-15.2443, -26.5854)
  spline S480 degree 3 poles (-63.5692, -23.3687) (-63.2352, -23.4038) (-62.9188, -23.4214) (-62.62, -23.4214) knots 0 0 0 0 1 1 1 1
  spline S481 degree 3 poles (-40.3091, -9.8821) (-41.1704, -9.4338) (-42.0581, -9.0955) (-42.9722, -8.8669) knots 0 0 0 0 1 1 1 1
  spline S482 degree 3 poles (-46.2944, -6.7576) (-45.9077, -6.5467) (-45.4418, -6.3841) (-44.8969, -6.2698) knots 0 0 0 0 1 1 1 1
  spline S483 degree 3 poles (-52.6619, -11.5959) (-52.1082, -10.5852) (-51.225, -9.7195) (-50.0121, -8.9988) knots 0 0 0 0 1 1 1 1
  spline S484 degree 3 poles (-68.4734, -20.9957) (-68.4909, -21.0308) (-68.5173, -21.066) (-68.5525, -21.1011) knots 0 0 0 0 1 1 1 1
  spline S485 degree 3 poles (-64.5711, -23.2105) (-64.2371, -23.2808) (-63.9031, -23.3335) (-63.5692, -23.3687) knots 0 0 0 0 1 1 1 1
  spline S486 degree 3 poles (-20.9922, -7.8123) (-20.1309, -7.3377) (-19.3003, -6.9378) (-18.5005, -6.6126) knots 0 0 0 0 1 1 1 1
  spline S487 degree 3 poles (-21.7832, -8.2605) (-21.5195, -8.1023) (-21.2559, -7.9529) (-20.9922, -7.8123) knots 0 0 0 0 1 1 1 1
  spline S488 degree 3 poles (-17.4195, -27.851) (-17.1822, -27.5522) (-16.9229, -27.2358) (-16.6417, -26.9018) knots 0 0 0 0 1 1 1 1
  spline S489 degree 3 poles (-16.589, -26.8227) (-16.4835, -26.6997) (-16.3868, -26.581) (-16.2989, -26.4668) knots 0 0 0 0 1 1 1 1
  line L228 (-15.2443, -26.5854) -> (-15.6398, -26.9809)
  spline S490 degree 3 poles (-157.676, -18.2271) (-157.3156, -18.649) (-156.9069, -19.0885) (-156.4499, -19.5455) knots 0 0 0 0 1 1 1 1
  line L229 (-50.0121, -8.9988) -> (-46.2944, -6.7576)
  spline S491 degree 3 poles (-67.656, -22.2349) (-67.2517, -22.4282) (-66.7771, -22.6128) (-66.2322, -22.7886) knots 0 0 0 0 1 1 1 1
  spline S492 degree 3 poles (-68.5525, -21.1011) (-68.5876, -21.1539) (-68.6184, -21.2022) (-68.6448, -21.2461) knots 0 0 0 0 1 1 1 1
  line L230 (-16.3253, -5.9666) -> (-16.2594, -5.9666)
  spline S493 degree 3 poles (-53.8353, -15.2213) (-53.6068, -13.8151) (-53.2156, -12.6066) (-52.6619, -11.5959) knots 0 0 0 0 1 1 1 1
  line L231 (-220.9793, -2.5389) -> (-2.5393, -2.5389)
  line L232 (-16.0353, -26.1372) -> (-14.9542, -24.7397)
  spline S494 degree 3 poles (-156.4499, -19.5455) (-156.0808, -19.897) (-155.6897, -20.2398) (-155.2766, -20.5738) knots 0 0 0 0 1 1 1 1
  spline S495 degree 3 poles (-49.0101, -25.0561) (-50.6097, -24.2124) (-51.8358, -23.083) (-52.6883, -21.668) knots 0 0 0 0 1 1 1 1
  line L233 (-68.6843, -21.3912) -> (-68.6843, -21.4175)
  spline S496 degree 3 poles (-68.6843, -21.4175) (-68.6843, -21.523) (-68.592, -21.6504) (-68.4075, -21.7998) knots 0 0 0 0 1 1 1 1
  line L234 (-220.9793, -30.4789) -> (-220.9793, -2.5389)
  spline S497 degree 3 poles (-53.9671, -16.9615) (-53.9671, -16.6627) (-53.9583, -16.3683) (-53.9407, -16.0783) knots 0 0 0 0 1 1 1 1
  spline S498 degree 3 poles (-22.5478, -8.7087) (-22.3018, -8.5681) (-22.0469, -8.4187) (-21.7832, -8.2605) knots 0 0 0 0 1 1 1 1
  arc A51 (-16.0353, -26.1372) -> (-16.2989, -26.4668) centre (-7.7235, -33.0568) ccw
  line L235 (-23.3388, -9.2361) -> (-22.5478, -8.7087)
  line L236 (-16.6285, -26.8623) -> (-16.589, -26.8227)
  spline S499 degree 3 poles (-17.2613, -28.3915) (-17.5338, -28.5761) (-17.6876, -28.5981) (-17.7227, -28.4574) knots 0 0 0 0 1 1 1 1
  spline S500 degree 3 poles (-157.5309, -8.7878) (-157.9001, -8.946) (-158.2297, -9.4119) (-158.5197, -10.1853) knots 0 0 0 0 1 1 1 1
  spline S501 degree 3 poles (-16.378, -27.6664) (-16.6944, -27.9653) (-16.9889, -28.207) (-17.2613, -28.3915) knots 0 0 0 0 1 1 1 1
  line L237 (-16.1671, -27.4555) -> (-16.2726, -27.561)
  spline S502 degree 3 poles (-17.7227, -28.4574) (-17.7579, -28.352) (-17.6568, -28.1498) (-17.4195, -27.851) knots 0 0 0 0 1 1 1 1
  spline S503 degree 3 poles (-70.9518, -12.3474) (-70.9694, -12.2946) (-70.9782, -12.2419) (-70.9782, -12.1892) knots 0 0 0 0 1 1 1 1
  spline S504 degree 3 poles (-42.9722, -8.8669) (-43.6225, -8.6912) (-44.2597, -8.5637) (-44.8838, -8.4846) knots 0 0 0 0 1 1 1 1
  spline S505 degree 3 poles (-38.1998, -11.5827) (-38.7447, -10.8972) (-39.4478, -10.3303) (-40.3091, -9.8821) knots 0 0 0 0 1 1 1 1
  spline S506 degree 3 poles (-18.5005, -6.6126) (-17.7008, -6.2874) (-17.0196, -6.0809) (-16.4571, -5.993) knots 0 0 0 0 1 1 1 1
  spline S507 degree 3 poles (-60.7347, -23.3027) (-60.1459, -23.2236) (-59.6581, -23.0611) (-59.2714, -22.815) knots 0 0 0 0 1 1 1 1
  spline S508 degree 3 poles (-153.9978, -21.4966) (-153.5935, -21.7427) (-153.2024, -21.9756) (-152.8245, -22.1953) knots 0 0 0 0 1 1 1 1
  spline S509 degree 3 poles (-68.6448, -21.2461) (-68.6711, -21.2901) (-68.6843, -21.3384) (-68.6843, -21.3912) knots 0 0 0 0 1 1 1 1
  spline S510 degree 3 poles (-59.1791, -22.5645) (-59.1527, -22.4326) (-59.1395, -22.2613) (-59.1395, -22.0503) knots 0 0 0 0 1 1 1 1
  spline S511 degree 3 poles (-62.62, -23.4214) (-61.952, -23.4214) (-61.3236, -23.3818) (-60.7347, -23.3027) knots 0 0 0 0 1 1 1 1
  spline S512 degree 3 poles (-155.2766, -20.5738) (-154.8635, -20.9078) (-154.4372, -21.2154) (-153.9978, -21.4966) knots 0 0 0 0 1 1 1 1
  spline S513 degree 3 poles (-52.6883, -21.668) (-53.5408, -20.253) (-53.9671, -18.6842) (-53.9671, -16.9615) knots 0 0 0 0 1 1 1 1
  spline S514 degree 3 poles (-59.2714, -22.815) (-59.2362, -22.7798) (-59.2055, -22.6963) (-59.1791, -22.5645) knots 0 0 0 0 1 1 1 1
  spline S515 degree 3 poles (-68.4075, -21.7998) (-68.2229, -21.9493) (-67.9724, -22.0943) (-67.656, -22.2349) knots 0 0 0 0 1 1 1 1
  line L238 (-68.4206, -20.7979) -> (-68.4206, -20.8902)
  arc A52 (-66.2322, -22.7886) -> (-64.5711, -23.2105) centre (-62.0796, -9.9191) ccw
  line L239 (-70.9782, -12.1892) -> (-70.9782, -12.031)
  spline S516 degree 3 poles (-70.9782, -12.031) (-70.9782, -11.6267) (-70.9518, -11.2575) (-70.8991, -10.9236) knots 0 0 0 0 1 1 1 1
  line L240 (-2.5393, -2.5389) -> (-2.5393, -30.4789)
  line L241 (-2.5393, -30.4789) -> (-220.9793, -30.4789)
  line L242 (-16.2594, -5.9666) -> (-16.1935, -5.9666)
  spline S517 degree 3 poles (-16.3912, -5.993) (-16.3648, -5.993) (-16.3429, -5.9842) (-16.3253, -5.9666) knots 0 0 0 0 1 1 1 1
  line L243 (-16.4571, -5.993) -> (-16.3912, -5.993)
  spline S518 degree 3 poles (-14.9542, -24.7397) (-14.6027, -24.3003) (-14.2687, -23.8521) (-13.9523, -23.395) knots 0 0 0 0 1 1 1 1
  spline S519 degree 3 poles (-50.3417, -17.357) (-50.2626, -17.8844) (-50.1439, -18.3941) (-49.9857, -18.8863) knots 0 0 0 0 1 1 1 1
  line L244 (-33.0583, -15.3268) -> (-33.0583, -15.3927)
  spline S520 degree 3 poles (-37.0133, -13.8107) (-37.2769, -12.9758) (-37.6724, -12.2331) (-38.1998, -11.5827) knots 0 0 0 0 1 1 1 1
  spline S521 degree 3 poles (-49.9594, -18.8863) (-49.8715, -19.1676) (-49.6386, -19.5059) (-49.2606, -19.9014) knots 0 0 0 0 1 1 1 1
  line L245 (-31.6707, -8.3132) -> (-28.3749, -6.573)
  line L246 (-50.4867, -15.195) -> (-50.4867, -15.4586)
  line L247 (-49.9857, -18.8863) -> (-49.9857, -18.8599)
  spline S522 degree 3 poles (-49.2606, -19.9014) (-48.8827, -20.2969) (-48.3949, -20.7144) (-47.7973, -21.1539) knots 0 0 0 0 1 1 1 1
  line L248 (-33.0583, -15.3927) -> (-33.0583, -15.4586)
  spline S523 degree 3 poles (-39.3863, -23.6191) (-38.8941, -23.4697) (-38.4459, -23.2193) (-38.0416, -22.8677) knots 0 0 0 0 1 1 1 1
  spline S524 degree 3 poles (-36.4596, -17.4625) (-36.4596, -17.2867) (-36.464, -17.1066) (-36.4728, -16.922) knots 0 0 0 0 1 1 1 1
  spline S525 degree 3 poles (-38.0416, -22.8677) (-37.5846, -22.4634) (-37.2066, -21.7603) (-36.9078, -20.7584) knots 0 0 0 0 1 1 1 1
  line L249 (-36.2223, -22.3667) -> (-39.94, -24.7925)
  spline S526 degree 3 poles (-49.9462, -11.1213) (-50.3065, -12.3781) (-50.4867, -13.736) (-50.4867, -15.195) knots 0 0 0 0 1 1 1 1
  spline S527 degree 3 poles (-40.0455, -6.5467) (-37.9713, -7.1619) (-36.2926, -8.2341) (-35.0094, -9.7634) knots 0 0 0 0 1 1 1 1
  spline S528 degree 3 poles (-47.7973, -21.1539) (-47.1469, -21.6285) (-46.4042, -22.0855) (-45.5693, -22.5249) knots 0 0 0 0 1 1 1 1
  spline S529 degree 3 poles (-41.9439, -23.7642) (-41.5923, -23.8169) (-41.2495, -23.8433) (-40.9156, -23.8433) knots 0 0 0 0 1 1 1 1
  spline S530 degree 3 poles (-45.5693, -22.5249) (-44.7343, -22.9644) (-43.8774, -23.3071) (-42.9985, -23.5532) knots 0 0 0 0 1 1 1 1
  spline S531 degree 3 poles (-44.8838, -8.4846) (-45.5078, -8.4055) (-46.0746, -8.366) (-46.5844, -8.366) knots 0 0 0 0 1 1 1 1
  spline S532 degree 3 poles (-33.7306, -19.4664) (-34.1788, -20.6089) (-35.0094, -21.5757) (-36.2223, -22.3667) knots 0 0 0 0 1 1 1 1
  spline S533 degree 3 poles (-46.5844, -8.366) (-47.0766, -8.366) (-47.4985, -8.3967) (-47.85, -8.4583) knots 0 0 0 0 1 1 1 1
  spline S534 degree 3 poles (-47.85, -8.4583) (-48.2016, -8.5198) (-48.4564, -8.6033) (-48.6146, -8.7087) knots 0 0 0 0 1 1 1 1
  spline S535 degree 3 poles (-33.0583, -15.6168) (-33.0583, -17.0406) (-33.2824, -18.3238) (-33.7306, -19.4664) knots 0 0 0 0 1 1 1 1
  spline S536 degree 3 poles (-50.4867, -15.7487) (-50.4691, -16.2936) (-50.4208, -16.8297) (-50.3417, -17.357) knots 0 0 0 0 1 1 1 1
  spline S537 degree 3 poles (-40.7837, -6.3357) (-40.6607, -6.3709) (-40.5288, -6.4061) (-40.3882, -6.4412) knots 0 0 0 0 1 1 1 1
  line L250 (-23.3388, -6.573) -> (-23.3388, -9.2361)
  spline S538 degree 3 poles (-35.0094, -9.7634) (-33.7262, -11.2927) (-33.0758, -13.1472) (-33.0583, -15.3268) knots 0 0 0 0 1 1 1 1
  line L251 (-49.9857, -18.8599) -> (-49.9594, -18.8863)
  spline S539 degree 3 poles (-39.94, -24.7925) (-40.6958, -25.3022) (-41.4517, -25.6714) (-42.2075, -25.8999) knots 0 0 0 0 1 1 1 1
  spline S540 degree 3 poles (-36.9078, -20.7584) (-36.609, -19.7564) (-36.4596, -18.6578) (-36.4596, -17.4625) knots 0 0 0 0 1 1 1 1
  spline S541 degree 3 poles (-36.5123, -16.3815) (-36.5826, -15.5026) (-36.7496, -14.6457) (-37.0133, -13.8107) knots 0 0 0 0 1 1 1 1
  spline S542 degree 3 poles (-48.6146, -8.7087) (-49.142, -9.0603) (-49.5858, -9.8645) (-49.9462, -11.1213) knots 0 0 0 0 1 1 1 1
  spline S543 degree 3 poles (-42.9985, -23.5532) (-42.647, -23.6411) (-42.2954, -23.7114) (-41.9439, -23.7642) knots 0 0 0 0 1 1 1 1
  line L252 (-33.0583, -15.4586) -> (-33.0583, -15.5377)
  spline S544 degree 3 poles (-41.9834, -6.1512) (-41.5879, -6.1863) (-41.188, -6.2479) (-40.7837, -6.3357) knots 0 0 0 0 1 1 1 1
  line L253 (-27.0038, -21.8921) -> (-27.0038, -8.3923)
  spline S545 degree 3 poles (-36.4728, -16.922) (-36.4815, -16.7374) (-36.4947, -16.5573) (-36.5123, -16.3815) knots 0 0 0 0 1 1 1 1
  spline S546 degree 3 poles (-10.9465, -22.3535) (-11.298, -22.7315) (-11.5793, -23.0259) (-11.7902, -23.2368) knots 0 0 0 0 1 1 1 1
  line L254 (-70.7145, -10.238) -> (-70.7145, -10.2117)
  line L255 (-27.0038, -8.3923) -> (-31.6707, -8.3132)
  spline S547 degree 3 poles (-40.3882, -6.4412) (-40.2476, -6.4764) (-40.1158, -6.5115) (-39.9927, -6.5467) knots 0 0 0 0 1 1 1 1
  spline S548 degree 3 poles (-40.9156, -23.8433) (-40.3882, -23.8433) (-39.8785, -23.7686) (-39.3863, -23.6191) knots 0 0 0 0 1 1 1 1
  line L256 (-39.9927, -6.5203) -> (-40.0455, -6.5467)
  line L257 (-33.0583, -15.5377) -> (-33.0583, -15.6168)
  line L258 (-28.3749, -6.573) -> (-23.3388, -6.573)
  line L259 (-50.4867, -15.4586) -> (-50.4867, -15.7487)
  spline S549 degree 3 poles (-70.8991, -10.9236) (-70.8464, -10.5896) (-70.7849, -10.3611) (-70.7145, -10.238) knots 0 0 0 0 1 1 1 1
  spline S550 degree 3 poles (-44.5014, -26.2426) (-45.2397, -26.2426) (-45.9824, -26.1416) (-46.7294, -25.9394) knots 0 0 0 0 1 1 1 1
  spline S551 degree 3 poles (-46.7294, -25.9394) (-47.4765, -25.7373) (-48.2367, -25.4428) (-49.0101, -25.0561) knots 0 0 0 0 1 1 1 1
  line L260 (-27.0038, -25.9262) -> (-27.0038, -21.8921)
  line L261 (-39.9927, -6.5467) -> (-39.9927, -6.5203)
  spline S552 degree 3 poles (-42.2075, -25.8999) (-42.9634, -26.1284) (-43.728, -26.2426) (-44.5014, -26.2426) knots 0 0 0 0 1 1 1 1
  spline S553 degree 3 poles (-43.1304, -6.0984) (-42.7612, -6.0984) (-42.3789, -6.116) (-41.9834, -6.1512) knots 0 0 0 0 1 1 1 1
  constraint collinear L0 L40
  constraint collinear L1 L45
extrude "Extrude2" cut sketch "Sketch4" against normal blind 3.175 contours L4 S5 S6 L8 L12 S13 S14 L16 S15 S16 S201 A21 S202 L104 L149 | S4 L5 L7 L9 L10 L11 S10 A1 L14 L18 L19 A2 L20 L21 S21 L22 S23 S24 L25 S25 S26 S27 L26 S28 S29 S32 L27 | S481 S504 S505 S519 S520 S521 L246 L247 S522 S523 S524 S525 S526 S528 S529 S530 S531 S533 S534 S536 L251 S540 S541 S542 S543 S545 S548 L259 | L231 L234 L240 L241
